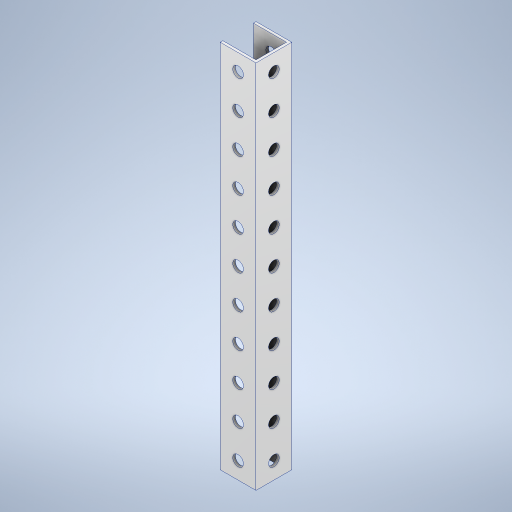
# Autodesk Inventor part: C-Channel 11in
Saved by Autodesk Inventor 2024 (Build 280153020, 153B)
## iProperties
Created: 2024-02-06
Part Number: C-Channel 11in
Material: Aluminum 6061
Document SubType Name: Modeling
Designer: scottst
Density: 2.7 g/cm^3
Appearance: Aluminum - Flat
Author: scottst
Autodesk Inventor part; units mm, degrees
ref_plane "YZ Plane" through (0, 0, 0) normal (1, 0, 0) x (0, 1, 0)
ref_plane "XZ Plane" through (0, 0, 0) normal (0, 1, 0) x (-1, 0, 0)
ref_plane "XY Plane" through (0, 0, 0) normal (0, 0, 1) x (1, 0, 0)
sketch "Sketch1" plane through (0, 0, 0) normal (0, 1, 0) x (-1, 0, 0)
  line L0 (-13.5, 13.5) -> (13.5, 13.5)
  line L1 (13.5, 13.5) -> (13.5, -13.5)
  line L2 (13.5, -13.5) -> (-13.5, -13.5)
  line L3 (-13.5, -13.5) -> (-13.5, 13.5)
  line L4 (-13.5, 13.5) -> (13.5, -13.5) construction
  line L5 (13.5, 13.5) -> (-13.5, -13.5) construction
  line L6 (11.5, -11.5) -> (11.5, 11.5)
  line L7 (11.5, 11.5) -> (-11.5, 11.5)
  line L8 (-11.5, 11.5) -> (-11.5, -11.5)
  line L9 (-11.5, -11.5) -> (11.5, -11.5)
  line L10 (11.5, 11.5) -> (13.5, 11.5)
  line L11 (11.5, -11.5) -> (13.5, -11.5)
  point P0 (0, 0)
  dimension "d0" = 27
  dimension "d1" = 27
  dimension "d2" = 2
  constraints: 24 end point, 4 parallel, 4 perpendicular, 2 midpoint, 2 point on line, 1 horizontal, 3 other
  measures "d0" distance of L1.end L2.end
  measures "d1" distance of L0.end L1.end
  measures "d2" distance between parallel lines of L1 L6
extrude "Extrusion1" add sketch "Sketch1" along normal blind 279.4 contours L0 L1 L10 L7 L8 L9 L11 L2 L3
sketch "Sketch2" plane through (-13.5, 0, 13.5) normal (0, 0, 1) x (1, 0, 0)
  line L0 (13.5, 0) -> (13.5, 12.7) construction
  circle A0 centre (13.5, 12.7) radius 4
  dimension "d5" = 12.7
  dimension "d6" = 8
  constraints: 2 end point, 1 centre point, 1 coincident, 1 vertical
  measures "d5" distance of L0.start L0.end
  measures "d6" diameter of A0
sketch "Sketch3" plane through (13.5, 0, 13.5) normal (1, 0, 0) x (0, 0, -1)
  line L0 (13.5, 0) -> (13.5, 12.7) construction
  circle A0 centre (13.5, 12.7) radius 4
  dimension "d7" = 12.7
  dimension "d8" = 8
  constraints: 2 end point, 1 centre point, 1 coincident, 1 vertical
  measures "d7" distance of L0.start L0.end
  measures "d8" diameter of A0
extrude "Extrusion2" cut sketch "Sketch2" against normal blind 93.1875
extrude "Extrusion3" cut sketch "Sketch3" against normal blind 117.95
pattern_linear "Rectangular Pattern1" count 11 spacing 25.4 along (0, 1, 0) of "Extrusion2", "Extrusion3"
body "Solid1"
